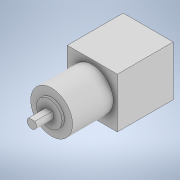
# Autodesk Inventor part: Stepper
Saved by Autodesk Inventor 2020 (Build 240168000, 168)
## iProperties
Created: 2020-05-15
Part Number: Stepper
Material: Generic
Document SubType Name: Modeling
Designer: jurre
Density: 1 g/cm^3
Appearance: Default
Author: jurre
Autodesk Inventor part; units mm, degrees
ref_plane "YZ Plane" through (0, 0, 0) normal (1, 0, 0) x (0, 1, 0)
ref_plane "XZ Plane" through (0, 0, 0) normal (0, 1, 0) x (-1, 0, 0)
ref_plane "XY Plane" through (0, 0, 0) normal (0, 0, 1) x (1, 0, 0)
sketch "Sketch1" plane through (0, 0, 0) normal (0, 0, 1) x (1, 0, 0)
  line L0 (-21.5, 21.5) -> (21.5, 21.5)
  line L1 (21.5, 21.5) -> (21.5, -21.5)
  line L2 (21.5, -21.5) -> (-21.5, -21.5)
  line L3 (-21.5, -21.5) -> (-21.5, 21.5)
  point P0 (0, 0)
  dimension "d0" = 43
  dimension "d1" = 43
  dimension "d2" = 21.5
  dimension "d3" = 21.5
  constraints: 8 end point, 2 parallel, 1 horizontal, 1 perpendicular
  measures "d0" distance of L0.start L0.end
  measures "d1" distance of L0.end L1.end
  measures "d2" distance from line of L1 point (0, 0)
  measures "d3" distance from line of L0 point (0, 0)
extrude "Extrusion1" add sketch "Sketch1" along normal blind 48
sketch "Sketch2" plane through (0, 0, 48) normal (0, 0, 1) x (1, 0, 0)
  circle A0 centre (0, 0) radius 18
  dimension "d6" = 36
  constraints: 1 centre point, 1 coincident
  measures "d6" diameter of A0
extrude "Extrusion2" add sketch "Sketch2" along normal blind 35
sketch "Sketch4" plane through (0, 0, 83) normal (0, 0, 1) x (1, 0, 0)
  circle A0 centre (0, 0) radius 11
  dimension "d9" = 22
  constraints: 1 centre point, 1 coincident
  measures "d9" diameter of A0
extrude "Extrusion3" add sketch "Sketch4" along normal blind 2
sketch "Sketch5" plane through (0, 0, 85) normal (0, 0, 1) x (1, 0, 0)
  circle A0 centre (0, 0) radius 4
  line L0 (0, -4) -> (0, 3) construction
  line L1 (0, 3) -> (-2.6458, 3)
  line L2 (0, 3) -> (2.6458, 3)
  dimension "d12" = 8
  dimension "d13" = 7
  constraints: 6 end point, 3 point on circle, 1 centre point, 1 coincident, 1 vertical
  measures "d12" diameter of A0
  measures "d13" distance of L0.start L0.end
extrude "Extrusion4" add sketch "Sketch5" along normal blind 15 contours A0 L1 L2 picked at (-0.1322, -1.6427)
body "Solid1"
